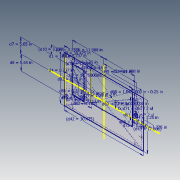
# Autodesk Inventor part: FLUGGER FRT COVER
Saved by Autodesk Inventor 2020.3 (Build 243373000, 373)
## iProperties
RuleStatus: InUse
AfterDocSave0: file://Part Number Cleaner
Created: 2020-01-03
Material: POLYCARBONATE, CLEAR
Vendor: HHMI: JRC - ID&F
Document SubType Name: Modeling
Designer: arnoldj
Density: 1.2 g/cm^3
Appearance: Polycarbonate (Clear)
DESIGN DEPARTMENT: HHMI: JRC - ID&F
ALTERED ITEM PART NUMBER: N/A
ALTERED ITEM VENDOR: N/A
ALTERED ITEM DESCRIPTION: N/A
Author: arnoldj
Revision Number: 0
Autodesk Inventor part; units mm, degrees
ref_plane "YZ Plane" through (0, 0, 0) normal (1, 0, 0) x (0, 1, 0)
ref_plane "XZ Plane" through (0, 0, 0) normal (0, 1, 0) x (-1, 0, 0)
ref_plane "XY Plane" through (0, 0, 0) normal (0, 0, 1) x (1, 0, 0)
sketch "Sketch1" plane through (0, 0, 0) normal (0, 0, 1) x (1, 0, 0)
  line L0 (0, 316.484) -> (0, -316.484) projected
  line L1 (-541.8455, 0) -> (541.8455, 0) projected
  line L2 (387.0325, -226.06) -> (-387.0325, -226.06)
  line L3 (-387.0325, -226.06) -> (-387.0325, 226.06)
  line L4 (-387.0325, 226.06) -> (387.0325, 226.06)
  line L5 (387.0325, 226.06) -> (387.0325, -226.06)
  line L6 (387.0325, -226.06) -> (-387.0325, 226.06) construction
  line L7 (-387.0325, -226.06) -> (387.0325, 226.06) construction
  line L8 (368.3127, -207.3402) -> (-368.3127, -207.3402) construction
  line L9 (-368.3127, -207.3402) -> (-368.3127, 207.3402) construction
  line L10 (-368.3127, 207.3402) -> (368.3127, 207.3402) construction
  line L11 (368.3127, 207.3402) -> (368.3127, -207.3402) construction
  line L12 (368.3127, -207.3402) -> (-368.3127, 207.3402) construction
  line L13 (-368.3127, -207.3402) -> (368.3127, 207.3402) construction
  line L14 (279.4, -72.39) -> (-127, -72.39)
  line L15 (-127, -72.39) -> (-127, 226.06)
  line L16 (-127, 226.06) -> (279.4, 226.06)
  line L17 (279.4, 226.06) -> (279.4, -72.39)
  line L18 (279.4, -72.39) -> (-127, 226.06) construction
  line L19 (-127, -72.39) -> (279.4, 226.06) construction
  point P0 (0, 0)
  point P1 (-304.4952, 207.3402)
  point P2 (0, 207.3402)
  point P3 (304.4952, 207.3402)
  point P4 (-304.4952, -207.3402)
  point P5 (0, -207.3402)
  point P6 (304.4952, -207.3402)
  point P7 (-368.3127, 143.51)
  point P8 (-368.3127, -143.51)
  point P9 (368.3127, 143.51)
  point P10 (368.3127, -117.0967)
  point P11 (76.2, 76.835)
  point P12 (-209.55, 207.3402)
  dimension "d0" = 774.065
  dimension "d1" = 452.12
  dimension "d3" = 18.7198
  dimension "d4" = 18.7198
  dimension "d5" = 304.4952
  dimension "d6" = 304.4952
  dimension "d7" = 143.51
  dimension "d8" = 143.51
  dimension "d9" = 82.5373
  dimension "d10" = 82.55
  dimension "d20" = 76.2
  dimension "d23" = 406.4
  dimension "d26" = 0
  dimension "d27" = 298.45
  dimension "d28" = 82.55
  dimension "d42" = 774.065
  dimension "d43" = 452.12
  constraints: 36 end point, 9 point on line, 8 midpoint, 6 parallel, 3 horizontal, 3 perpendicular, 2 vertical alignment, 1 horizontal alignment
  measures "d0" distance of L3.end L4.end
  measures "d1" distance of L2.end L3.end
  measures "d3" distance between parallel lines of L10 L4
  measures "d4" distance between parallel lines of L9 L3
  measures "d5" distance from line of L0 point (304.495, 207.34)
  measures "d6" distance from line of L0 point (-304.495, 207.34)
  measures "d7" distance from line of L1 point (-368.313, 143.51)
  measures "d8" distance from line of point (-368.313, -143.51) L1
  measures "d9" distance from line of point (-304.495, 207.34) L3
  measures "d10" distance from line of point (-368.313, 143.51) L4
  measures "d20" distance from line of L0 point (76.2, 76.835)
  measures "d23" distance of L15.end L16.end
  measures "d26" distance between parallel lines of L16 L4
  measures "d27" distance of L14.end L15.end
  measures "d28" distance from line of point (-209.55, 207.34) L15
  measures "d42" distance of L2.start L2.end
  measures "d43" distance of L4.end L2.start
extrude "Extrusion1" add sketch "Sketch1" against normal blind 6.35
hole "Hole1-M6 Clearance" at (-304.4952, 207.3402, 0) at (304.4952, 207.3402, 0) at (-304.4952, -207.3402, 0) at (0, -207.3402, 0) at (304.4952, -207.3402, 0) at (-368.3127, 143.51, 0) at (-368.3127, -143.51, 0) at (368.3127, 143.51, 0) at (368.3127, -117.0967, 0) at (-209.55, 207.3402, 0) direction (0, 0, -1) diameter 7.9375 end through all
extrude "Extrusion2" cut sketch "Sketch1" against normal up to next contours L4 L17 L1 L0 | L0 L1 L15 L4 | L1 L17 L14 L0 | L0 L14 L15 L1
sketch "Sketch3" plane through (0, 0, 0) normal (0, 0, 1) x (1, 0, 0)
  line L0 (0, 285.75) -> (0, -132.08) projected
  line L1 (-520.319, 0) -> (412.6865, 0) projected
  line L2 (-127, -72.39) -> (279.4, -72.39) projected
  line L3 (-387.0325, 226.06) -> (-127, 226.06) projected
  point P0 (0, 0)
  point P1 (-156.9974, -53.34)
  point P2 (-156.9974, -25.34)
  point P3 (-156.9974, 179.01)
  point P4 (-156.9974, 207.01)
  dimension "d29" = 28
  dimension "d30" = 28
  dimension "d31" = 156.9974
  dimension "d39" = 19.05
  dimension "d40" = 19.05
  dimension "d44" = 204.35
  constraints: 3 vertical alignment
  measures "d29" distance of point (-156.997, -25.34) point (-156.997, -53.34)
  measures "d30" distance of point (-156.997, 207.01) point (-156.997, 179.01)
  measures "d31" distance from line of point (-156.997, -53.34) L0
  measures "d39" distance from line of L2 point (-156.997, -53.34)
  measures "d40" distance from line of point (-156.997, 207.01) L3
  measures "d44" distance of point (-156.997, -25.34) point (-156.997, 179.01)
hole "Hole2-Tap M5" at (-156.9974, -53.34, 0) at (-156.9974, -25.34, 0) at (-156.9974, 179.01, 0) at (-156.9974, 207.01, 0) direction (0, 0, -1) diameter 4.064 end through all
fillet "Fillet1" radius 6.35 6 edges at (279.4, 226.06, -3.175) (-127, 226.06, -3.175) (-387.0325, 226.06, -3.175) (-387.0325, -226.06, -3.175) (387.0325, -226.06, -3.175) (387.0325, 226.06, -3.175)
sketch "Sketch4" plane through (0, 0, 0) normal (0, 0, 1) x (1, 0, 0)
  line L0 (0, 285.75) -> (0, -132.08) projected
  line L1 (-541.8455, 0) -> (541.8455, 0) projected
  line L2 (279.4, -72.39) -> (279.4, 219.71) construction
  line L3 (285.75, 172.085) -> (279.4, 172.085)
  line L4 (279.4, 172.085) -> (279.4, -31.115)
  line L5 (279.4, -31.115) -> (285.75, -31.115)
  line L6 (285.75, -31.115) -> (285.75, 172.085)
  line L7 (285.75, 172.085) -> (279.4, -31.115) construction
  line L8 (279.4, 172.085) -> (285.75, -31.115) construction
  line L9 (285.75, 226.06) -> (380.6825, 226.06) projected
  line L10 (-387.0325, 226.06) -> (387.0325, 226.06) projected
  line L11 (331.31, 172.085) -> (299.56, 172.085) construction
  line L12 (299.56, 172.085) -> (299.56, -31.115) construction
  line L13 (299.56, -31.115) -> (331.31, -31.115) construction
  line L14 (331.31, -31.115) -> (331.31, 172.085) construction
  line L15 (331.31, 172.085) -> (299.56, -31.115) construction
  line L16 (299.56, 172.085) -> (331.31, -31.115) construction
  circle A0 centre (316.7126, 45.085) radius 15.875
  point P0 (0, 0)
  point P1 (282.575, 70.485)
  point P2 (282.575, 70.485)
  point P3 (76.2, 76.835)
  point P4 (315.435, 70.485)
  dimension "d48" = 6.35
  dimension "d61" = 203.2
  dimension "d68" = 20.16
  dimension "d69" = 70.485
  dimension "d71" = 101.6
  dimension "d72" = 31.75
  dimension "d73" = 203.2
  dimension "d94" = 31.75
  dimension "d95" = 316.7126
  dimension "d96" = 45.085
  constraints: 24 end point, 5 midpoint, 4 coincident, 4 parallel, 2 horizontal, 2 perpendicular, 1 centre point, 1 point on line, 1 vertical alignment
  measures "d48" distance of L4.end L5.end
  measures "d61" distance of point (299.56, 172.085) L12.end
  measures "d68" distance from line of L2 point (299.56, 172.085)
  measures "d69" distance from line of point (282.575, 70.485) L1
  measures "d71" vertical distance of point (282.575, 70.485) point (299.56, 172.085)
  measures "d72" distance of L12.end L13.end
  measures "d73" distance of L5.end L3.start
  measures "d94" diameter of A0
  measures "d95" distance from line of A0.centre L0
  measures "d96" distance from line of A0.centre L1
extrude "Extrusion3" cut sketch "Sketch4" against normal up to next contours L4 L3 L6 L1 | L1 L6 L5 L4
hole "Hole3-Tap M5" at (299.56, -31.115, 0) at (299.56, 172.085, 0) at (331.31, -31.115, 0) at (331.31, 172.085, 0) direction (0, 0, -1) diameter 4.064 end through all
fillet "Fillet2" radius 3.175 4 edges at (279.4, -31.115, -3.175) (285.75, -31.115, -3.175) (285.75, 172.085, -3.175) (279.4, 172.085, -3.175)
sketch "Sketch5" plane through (0, 0, -6.35) normal (0, 0, -1) x (-1, 0, 0)
  line L0 (0, -316.484) -> (0, 316.484) projected
  line L1 (-541.8455, 0) -> (541.8455, 0) projected
  line L2 (199.898, 161.925) -> (314.198, 161.925)
  line L3 (314.198, 161.925) -> (314.198, -98.425)
  line L4 (314.198, -98.425) -> (199.898, -98.425)
  line L5 (199.898, -98.425) -> (199.898, 161.925)
  line L6 (199.898, 161.925) -> (314.198, -98.425) construction
  line L7 (314.198, 161.925) -> (199.898, -98.425) construction
  line L8 (368.3127, -207.3402) -> (368.3127, 207.3402) construction
  line L9 (387.0325, -219.71) -> (387.0325, 219.71) projected
  line L10 (127, 219.71) -> (127, -72.39) projected
  line L11 (193.548, 168.275) -> (320.548, 168.275) construction
  line L12 (320.548, 168.275) -> (320.548, -104.775) construction
  line L13 (320.548, -104.775) -> (193.548, -104.775) construction
  line L14 (193.548, -104.775) -> (193.548, 168.275) construction
  line L15 (193.548, 168.275) -> (320.548, -104.775) construction
  line L16 (320.548, 168.275) -> (193.548, -104.775) construction
  line L17 (320.548, 31.75) -> (193.548, 31.75) construction
  line L18 (193.548, 50.8) -> (320.548, 50.8) construction
  line L19 (320.548, 50.8) -> (320.548, 12.7) construction
  line L20 (320.548, 12.7) -> (193.548, 12.7) construction
  line L21 (193.548, 12.7) -> (193.548, 50.8) construction
  line L22 (193.548, 50.8) -> (320.548, 12.7) construction
  line L23 (320.548, 50.8) -> (193.548, 12.7) construction
  point P0 (0, 0)
  point P1 (257.048, 31.75)
  point P2 (304.4952, 207.3402)
  dimension "d74" = 114.3
  dimension "d75" = 260.35
  dimension "d76" = 257.048
  dimension "d77" = 31.75
  dimension "d78" = 45.4152
  dimension "d79" = 129.9845
  dimension "d80" = 130.048
  dimension "d81" = 6.35
  dimension "d82" = 6.35
  dimension "d83" = 19.05
  constraints: 38 end point, 8 coincident, 8 midpoint, 6 parallel, 3 horizontal, 3 perpendicular, 1 point on line
  measures "d74" distance of L3.end L4.end
  measures "d75" distance of L4.end L2.start
  measures "d76" distance from line of L0 point (257.048, 31.75)
  measures "d77" distance from line of L1 point (257.048, 31.75)
  measures "d78" distance from line of point (304.495, 207.34) L2
  measures "d79" distance from line of L9 point (257.048, 31.75)
  measures "d80" distance from line of L10 point (257.048, 31.75)
  measures "d81" distance between parallel lines of L12 L3
  measures "d82" distance between parallel lines of L13 L4
  measures "d83" distance between parallel lines of L20 L17
hole "Hole4" at (-320.548, -104.775, -6.35) at (-193.548, -104.775, -6.35) at (-193.548, 12.7, -6.35) at (-193.548, 50.8, -6.35) at (-320.548, 50.8, -6.35) at (-320.548, 12.7, -6.35) at (-320.548, 168.275, -6.35) at (-193.548, 168.275, -6.35) direction (0, 0, 1) diameter 4.134 end through all thread size "M5x0.8" class "6H" standard "ANSI Metric M Profile"
extrude "Extrusion4" cut sketch "Sketch5" against normal through all
fillet "Fillet3" radius 3.175 4 edges at (-199.898, -98.425, -3.175) (-314.198, -98.425, -3.175) (-314.198, 161.925, -3.175) (-199.898, 161.925, -3.175)
extrude "Extrusion5" cut sketch "Sketch4" against normal through all contours A0
equation "\"d71\" = 0.5 * d61"
body "Solid1"
